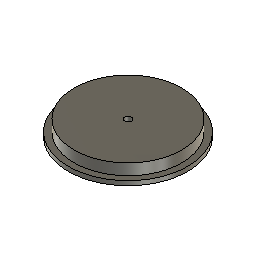
fan_plug (Autodesk Fusion 360 design; units mm, degrees)
part number: 2026-08-22-19-59-32-965
Autodesk Fusion 360 part; units mm, degrees
sketch "Flange" plane through (0, 0, 0) normal (0, 0, 1) x (1, 0, 0)
  circle A0 centre (0, 0) radius 21.5
extrude "Flange (1)" add sketch "Flange" along normal blind 1.6
ref_plane "WorkPlane1" through (0, 0, 1.6) normal (0, 0, 1) x (1, 0, 0)
sketch "Press-fit body" plane through (0, 0, 1.6) normal (0, 0, 1) x (1, 0, 0)
  circle A0 centre (0, 0) radius 19.35
extrude "Press-fit body (1)" add sketch "Press-fit body" along normal blind 4
sketch "Puller pilot" plane through (0, 0, 0) normal (0, 0, 1) x (1, 0, 0)
  circle A0 centre (0, 0) radius 1.25
extrude "Puller pilot (1)" cut sketch "Puller pilot" along normal mid plane 11.2
named bodies: "Fan Plug"
